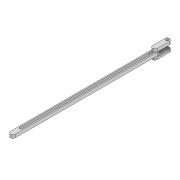
# Autodesk Inventor part: Part_6
Saved by Autodesk Inventor 2022 (Build 260153000, 153)
## iProperties
Created: 2022-04-22
Part Number: Part_6
Material: Generic
Document SubType Name: Modeling
Designer: dell
Density: 1 g/cm^3
Appearance: Default
Author: dell
Autodesk Inventor part; units mm, degrees
ref_plane "YZ Plane" through (0, 0, 0) normal (1, 0, 0) x (0, 1, 0)
ref_plane "XZ Plane" through (0, 0, 0) normal (0, 1, 0) x (-1, 0, 0)
ref_plane "XY Plane" through (0, 0, 0) normal (0, 0, 1) x (1, 0, 0)
sketch "Sketch1" plane through (0, 0, 0) normal (0, 1, 0) x (-1, 0, 0)
  line L0 (0, 0) -> (0, -189.937) construction
  line L1 (3, 0) -> (3, -189.937)
  line L2 (-3, -189.937) -> (-3, 0)
  arc A0 (3, 0) -> (-3, 0) centre (0, 0) ccw
  arc A1 (-3, -189.937) -> (3, -189.937) centre (0, -189.937) ccw
  circle A2 centre (0, -189.937) radius 1.6
  line L3 (0, -10) -> (0, -169.937) construction
  line L4 (-1.6, -10) -> (-1.6, -169.937)
  line L5 (1.6, -169.937) -> (1.6, -10)
  arc A3 (1.6, -10) -> (-1.6, -10) centre (0, -10) ccw
  arc A4 (-1.6, -169.937) -> (1.6, -169.937) centre (0, -169.937) ccw
  point P0 (0, -94.9685)
  point P1 (0, -89.9685)
  dimension "d1" = 3.2
  dimension "d2" = 6
  dimension "d3" = 189.937
  dimension "d16" = 3.2
  dimension "d17" = 20
  dimension "d18" = 10
  constraints: 16 end point, 8 point on circle, 8 tangent, 5 centre point, 2 midpoint, 2 parallel, 2 point on line, 1 coincident, 1 vertical
  measures "d1" diameter of A2
  measures "d2" distance between parallel lines of L2 L1
  measures "d3" distance of L0.end L0.start
  measures "d16" diameter of A4
  measures "d17" distance of L0.end L3.end
  measures "d18" distance of L0.start L3.start
extrude "Extrusion1" add sketch "Sketch1" along normal blind 4
sketch "Sketch2" plane through (0, 4, 0) normal (0, 1, 0) x (1, 0, 0)
  line L0 (-3, 189.937) -> (-3, 0) projected
  arc A0 (-3, 0) -> (3, 0) centre (0, 0) ccw projected
  line L1 (3, 0) -> (3, 189.937) projected
  arc A1 (3, 189.937) -> (-3, 189.937) centre (0, 189.937) ccw projected
  arc A2 (-1.6, 10) -> (1.6, 10) centre (0, 10) ccw projected
  line L2 (-1.6, 10) -> (-1.6, 169.937) projected
  arc A3 (1.6, 169.937) -> (-1.6, 169.937) centre (0, 169.937) ccw projected
  line L3 (1.6, 169.937) -> (1.6, 10) projected
  circle A4 centre (0, 189.937) radius 1.6 projected
  line L4 (-3, 189.937) -> (-3, 0) projected
  line L5 (3, 0) -> (3, 189.937) projected
  circle A5 centre (0, 174.937) radius 3
  point P0 (-3, 174.937)
  point P1 (3, 174.937)
  dimension "d20" = 15
  dimension "d21" = 6
  constraints: 1 centre point, 1 tangent
  measures "d20" distance of A1.centre A5.centre
  measures "d21" diameter of A5
extrude "Extrusion2" add sketch "Sketch2" along normal blind 4 contours A1 L1 A5 L0 | A5
sketch "Sketch3" plane through (0, 0, 0) normal (0, -1, 0) x (1, 0, 0)
  line L0 (-3, -189.937) -> (-3, 0) projected
  arc A0 (-3, -189.937) -> (3, -189.937) centre (0, -189.937) ccw projected
  line L1 (3, 0) -> (3, -189.937) projected
  arc A1 (3, 0) -> (-3, 0) centre (0, 0) ccw projected
  arc A2 (1.6, -10) -> (-1.6, -10) centre (0, -10) ccw projected
  line L2 (1.6, -169.937) -> (1.6, -10) projected
  arc A3 (-1.6, -169.937) -> (1.6, -169.937) centre (0, -169.937) ccw projected
  line L3 (-1.6, -10) -> (-1.6, -169.937) projected
  circle A4 centre (0, -189.937) radius 1.6 projected
  circle A5 centre (0, -174.937) radius 3
  point P0 (3, -174.937)
  point P1 (-3, -174.937)
  dimension "d24" = 6
  dimension "d25" = 15
  constraints: 1 centre point
  measures "d24" diameter of A5
  measures "d25" distance of A0.centre A5.centre
extrude "Extrusion3" add sketch "Sketch3" along normal blind 4 contours L0 A5 L1 A0 | A5
extrude "Extrusion4" cut sketch "Sketch2" against normal blind 5 contours A1 L1 A5 L0
sketch "Sketch4" plane through (0, -1, 0) normal (0, 1, 0) x (1, 0, 0)
  line L0 (-3, 174.937) -> (-3, 189.937) projected
  arc A0 (3, 174.937) -> (-3, 174.937) centre (0, 174.937) ccw projected
  line L1 (3, 189.937) -> (3, 174.937) projected
  arc A1 (3, 189.937) -> (-3, 189.937) centre (0, 189.937) ccw projected
  circle A2 centre (0, 189.937) radius 1.6 projected
  point P0 (0, 0)
extrude "Extrusion5" cut sketch "Sketch4" against normal blind 0.2
sketch "Sketch5" plane through (0, 4, 0) normal (0, -1, 0) x (1, 0, 0)
  line L0 (-3, -189.937) -> (-3, -174.937) projected
  arc A0 (-3, -189.937) -> (3, -189.937) centre (0, -189.937) ccw projected
  line L1 (3, -174.937) -> (3, -189.937) projected
  arc A1 (-3, -174.937) -> (3, -174.937) centre (0, -174.937) ccw projected
  circle A2 centre (0, -189.937) radius 1.6 projected
  point P0 (0, 0)
extrude "Extrusion6" cut sketch "Sketch5" against normal blind 0.2
body "Solid1"
